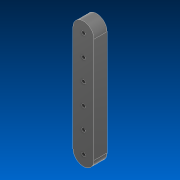
# Autodesk Inventor part: Motor Bracket Seperator
Saved by Autodesk Inventor 2022.2 (Build 262287000, 287)
## iProperties
Created: 2022-03-21
Part Number: Motor Bracket Seperator
Material: PET Plastic
Document SubType Name: Modeling
Designer: omard
Density: 1.541 g/cm^3
Appearance: Smooth - Black
Author: omard
Autodesk Inventor part; units mm, degrees
ref_plane "YZ Plane" through (0, 0, 0) normal (1, 0, 0) x (0, 1, 0)
ref_plane "XZ Plane" through (0, 0, 0) normal (0, 1, 0) x (-1, 0, 0)
ref_plane "XY Plane" through (0, 0, 0) normal (0, 0, 1) x (1, 0, 0)
sketch "Sketch1" plane through (0, 0, 0) normal (0, 0, 1) x (1, 0, 0)
  line L0 (0, -63.5) -> (0, 63.5) construction
  line L1 (12.7, -63.5) -> (12.7, 63.5)
  line L2 (-12.7, 63.5) -> (-12.7, -63.5)
  arc A0 (-12.7, -63.5) -> (12.7, -63.5) centre (0, -63.5) ccw
  arc A1 (12.7, 63.5) -> (-12.7, 63.5) centre (0, 63.5) ccw
  point P0 (0, 0)
  point P1 (0, 38.1)
  point P2 (0, 12.7)
  point P3 (0, -12.7)
  point P4 (0, -38.1)
  dimension "d0" = 63.5
  dimension "d1" = 25.4
  dimension "d2" = 25.4
  dimension "d3" = 25.4
  dimension "d4" = 25.4
  dimension "d5" = 25.4
  constraints: 8 end point, 4 point on circle, 4 point on line, 4 tangent, 2 centre point, 2 coincident, 1 midpoint, 1 parallel, 1 vertical
  measures "d0" distance of point (0, 0) L0.end
  measures "d1" diameter of A1
  measures "d2" distance of point (0, 63.5) point (0, 38.1)
  measures "d3" distance of point (0, 12.7) point (0, 38.1)
  measures "d4" distance of point (0, -38.1) point (0, -63.5)
  measures "d5" distance of point (0, -12.7) point (0, -38.1)
extrude "Extrusion1" add sketch "Sketch1" along normal blind 15.875
hole "Hole1" at (0, 38.1, 0) at (0, 12.7, 0) at (0, -12.7, 0) at (0, -38.1, 0) at (0, -63.5, 0) at (0, 63.5, 0) direction (0, 0, 1) diameter 4.318 end through all start extended yes
body "Solid1"
